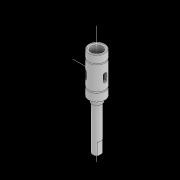
# Autodesk Inventor part: iner_sleeve
Saved by Autodesk Inventor 2021 (Build 250183000, 183)
## iProperties
Created: 2024-02-18
Part Number: iner_sleeve
Material: Generic
Document SubType Name: Modeling
Designer: top10
Density: 1 g/cm^3
Appearance: Default
Mass: 0.54823 g
Surface Area: 9.47924 cm^2
Volume: 0.54823 cm^3
Author: top10
Autodesk Inventor part; units mm, degrees
sketch "Sketch1" plane through (0, 0, 0) normal (0, 0, 1) x (1, 0, 0)
  line L0 (0, 6.8765) -> (0, -6.8765)
  line L1 (2.75, 0) -> (4, 0)
  line L2 (4, -20) -> (0, -20)
  line L3 (2.75, 0) -> (2.75, -16)
  line L4 (2.75, -16) -> (0, -16)
  line L5 (0, -16) -> (0, -20)
  line L6 (-11.1246, -10.5) -> (11.1246, -10.5)
  line L7 (4, 0) -> (4, -4.956)
  line L8 (4, 0) -> (4, -20)
  circle A0 centre (4, -16) radius 0.25
  circle A1 centre (4, -4) radius 0.25
  point P0 (0, 0)
  point P1 (0, 0)
  point P2 (0, -10.5)
  point P3 (4, -10.5)
  point P4 (4, -16.25)
  point P5 (4, -15.75)
  point P6 (4, -4.25)
  point P7 (4, -3.75)
  point P8 (4, -4.25)
  point P9 (4, -3.75)
  dimension "d2" = 20
  dimension "d5" = 5.5
  dimension "d6" = 16
  dimension "d8" = 10.5
  dimension "d63" = 8
  dimension "d66" = 0.5
  dimension "d81" = 4
  dimension "d82" = 16
  constraints: 18 end point, 4 perpendicular, 4 point on line, 3 vertical, 2 centre point, 2 horizontal, 2 midpoint, 2 vertical alignment, 1 coincident, 1 equal radius, 1 horizontal alignment, 1 parallel
  measures "d2" distance of L1.end L2.start
  measures "d5" diameter of L3 L0
  measures "d6" distance between parallel lines of L1 L4
  measures "d8" distance of point (0, -10.5) point (0, 0)
  measures "d63" diameter of L8 L0
  measures "d66" diameter of A0
  measures "d81" distance of L1.end A1.centre
  measures "d82" distance of L1.end A0.centre
revolve "Revolution1" add sketch "Sketch1" angle 360 about axis through (0, 6.8765, 0) along (0, -1, 0) contours L1 L7 A1 L8 L6 L3 | L6 L8 A0 L2 L5 L4 L3
ref_plane "Work Plane1" through (4, -10.5, 0) normal (1, 0, 0) x (0, 1, 0)
sketch "Sketch2" plane through (4, -10.5, 0) normal (1, 0, 0) x (0, 1, 0)
  line L0 (-1.25, 0) -> (1.25, 0) construction
  line L1 (-1.25, -1) -> (1.25, -1)
  line L2 (1.25, 1) -> (-1.25, 1)
  arc A0 (-1.25, 1) -> (-1.25, -1) centre (-1.25, 0) ccw
  arc A1 (1.25, -1) -> (1.25, 1) centre (1.25, 0) ccw
  point P0 (10.5, 0)
  point P1 (0, 0)
  point P2 (0, 0)
  dimension "d9" = 2
  dimension "d10" = 2.5
  constraints: 8 end point, 4 point on circle, 4 tangent, 2 centre point, 1 coincident, 1 horizontal, 1 midpoint, 1 parallel
  measures "d9" distance between parallel lines of L2 L1
  measures "d10" distance of L0.start L0.end
extrude "Extrusion1" [suppressed]
chamfer "Chamfer1" distance 0.5 angle 45 1 edges at (-2.75, 0, 0)
pattern_circular "Circular Pattern1" [suppressed]
ref_plane "Work Plane2" through (0, 0, 0) normal (1, 0, 0) x (0, 1, 0)
sketch "Sketch3" plane through (0, 0, 0) normal (1, 0, 0) x (0, 1, 0)
  line L0 (0.427, -0.05) -> (-18.843, -0.05)
  line L1 (-18.843, -0.05) -> (-18.843, 0.05)
  line L2 (-18.843, 0.05) -> (0.427, 0.05)
  line L3 (0.427, 0.05) -> (0.427, -0.05)
  line L4 (-16, 2.75) -> (-16, -2.75) projected
  point P0 (0, 0)
  point P1 (-18.843, 0)
  point P2 (-16, 0)
  point P3 (-16, 0.05)
  point P4 (-16, -0.05)
  dimension "d20" = 0.1
  constraints: 8 end point, 2 midpoint, 2 parallel, 1 horizontal, 1 horizontal alignment, 1 perpendicular
  measures "d20" distance between parallel lines of L0 L2
extrude "Extrusion2" [suppressed]
feature "Unwrap1" [suppressed]
sketch "Sketch5" plane through (0, -20, 0) normal (0, -1, 0) x (1, 0, 0)
  circle A0 centre (0, 0) radius 2.5
  point P0 (0, 0)
  dimension "d28" = 5
  constraints: 1 centre point, 1 coincident
  measures "d28" diameter of A0
extrude "Extrusion4" add sketch "Sketch5" along normal blind 2.5
sketch "Sketch6" plane through (0, -22.5, 0) normal (0, -1, 0) x (1, 0, 0)
  circle A0 centre (0, 0) radius 2
  point P0 (0, 0)
  dimension "d33" = 4
  constraints: 1 centre point, 1 coincident
  measures "d33" diameter of A0
extrude "Extrusion5" add sketch "Sketch6" along normal blind 22
sketch "Sketch7" plane through (0, 0, 0) normal (0, 0, 1) x (1, 0, 0)
  line L0 (-2, -22.5) -> (-2, -44.5) projected
  line L1 (-2.5, -22.5) -> (2.5, -22.5) projected
  arc A0 (-2, -22.75) -> (-2, -22.5) centre (-2, -22.625) ccw
  line L2 (0, 8.9) -> (0, -53.4) projected
  point P0 (0, 0)
  dimension "d42" = 0.25
  constraints: 3 point on line, 2 point on circle, 1 centre point, 1 tangent
  measures "d42" diameter of A0
revolve "Revolution2" cut sketch "Sketch7" angle 360 about axis through (0, -8, 0) along (0, -1, 0)
sketch "Sketch8" plane through (0, 0, 0) normal (1, 0, 0) x (0, 1, 0)
  line L0 (-20, 4) -> (-20, -4) projected
  circle A0 centre (-4, 0) radius 0.25
  circle A1 centre (-16, 0) radius 0.25
  line L1 (-16.25, 4) -> (-16.25, -4) projected
  line L2 (-15.75, 4) -> (-15.75, -4) projected
  line L3 (-4.25, 4) -> (-4.25, -4) projected
  line L4 (-3.75, 4) -> (-3.75, -4) projected
  point P0 (0, 0)
  constraints: 4 tangent, 2 centre point, 2 horizontal alignment
extrude "Extrusion6" cut sketch "Sketch8" against normal blind 10
chamfer "Chamfer4" distance 0.25 angle 45 1 edges at (-2, -44.5, 0)
sketch "Sketch10" plane through (0, 0, 0) normal (1, 0, 0) x (0, 1, 0)
  line L0 (-26.4, 2) -> (-26.9, 2)
  line L1 (-26.9, 2) -> (-26.9, 1.5)
  line L2 (-26.9, 1.5) -> (-26.4, 1.5)
  line L3 (-26.4, 1.5) -> (-26.4, 2)
  line L4 (-22.75, 2) -> (-44.25, 2) projected
  line L5 (-22.5, 2.5) -> (-22.5, -2.5) projected
  line L6 (-22.5, 0) -> (-23.5282, 0)
  point P0 (0, 0)
  dimension "d57" = 0.5
  dimension "d70" = 4.4
  dimension "d71" = 3
  constraints: 10 end point, 2 horizontal, 2 parallel, 1 midpoint, 1 perpendicular, 1 point on line
  measures "d57" distance of L0.start L0.end
  measures "d70" distance from line of L5 L1.end
  measures "d71" diameter of L2 L6
revolve "Revolution3" [suppressed]
chamfer "Chamfer5" distance 0.25 angle 45 1 edges at (-4, 0, 0)
ref_plane "Work Plane3" through (0, 0, 0) normal (0, 1, 0) x (1, 0, 0)
sketch "Sketch11" plane through (0, 0, 0) normal (0, 1, 0) x (1, 0, 0)
  point P0 (0, 0)
  point P1 (-4.4001, -3.2008)
hole "Hole1" at (0, 0, 0) direction (0, -1, 0) diameter 5.5 depth 18 tip angle 118
sketch "Sketch12" plane through (0, 0, 0) normal (0, 0, 1) x (1, 0, 0)
  line L0 (2, -44.5) -> (1.5, -44.5)
  line L1 (1.5, -44.5) -> (1.5, -38.5)
  line L2 (1.5, -38.5) -> (2, -38.5)
  line L3 (2, -38.5) -> (2, -44.5)
  line L4 (1.75, -44.5) -> (-1.75, -44.5) projected
  line L5 (2, -22.75) -> (2, -44.25) projected
  point P0 (0, 0)
  dimension "d83" = 0.5
  dimension "d84" = 6
  constraints: 8 end point, 2 parallel, 1 horizontal, 1 midpoint, 1 perpendicular, 1 point on line
  measures "d83" distance between parallel lines of L3 L1
  measures "d84" distance between parallel lines of L0 L2
extrude "Extrusion8" cut sketch "Sketch12" against normal mid plane 10
ref_plane "Work Plane4" through (4, -10.5, 0) normal (1, 0, 0) x (0, 1, 0)
sketch "Sketch13" plane through (4, -10.5, 0) normal (1, 0, 0) x (0, 1, 0)
  line L0 (1.33, 0) -> (-1.33, 0) construction
  line L1 (1.33, 0.8) -> (-1.33, 0.8)
  line L2 (-1.33, -0.8) -> (1.33, -0.8)
  arc A0 (1.33, -0.8) -> (1.33, 0.8) centre (1.33, 0) ccw
  arc A1 (-1.33, 0.8) -> (-1.33, -0.8) centre (-1.33, 0) ccw
  point P0 (10.5, 0)
  point P1 (0, 0)
  point P2 (0, 0)
  dimension "d90" = 2.66
  dimension "d91" = 1.6
  constraints: 8 end point, 4 point on circle, 4 tangent, 2 centre point, 1 coincident, 1 horizontal, 1 midpoint, 1 parallel
  measures "d90" distance of L2.start L2.end
  measures "d91" distance between parallel lines of L2 L1
extrude "Extrusion9" cut sketch "Sketch13" against normal up to surface
pattern_circular "Circular Pattern2" count 3 over 360 about axis through (0, 6.8765, 0) along (0, -1, 0) of "Extrusion9"
body "Solid1"
body "Srf1"
